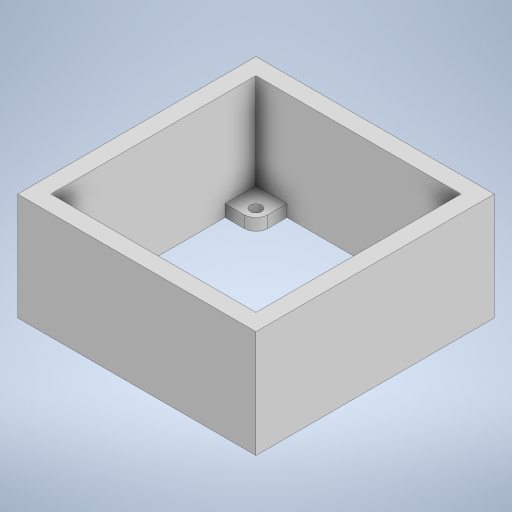
# Autodesk Inventor part: BigMotorDerzavka
Saved by Autodesk Inventor 2024 (Build 280153000, 153)
## iProperties
Created: 2023-11-07
Part Number: BigMotorDerzavka
Material: Generic
Document SubType Name: Modeling
Designer: KirikDK
Density: 1 g/cm^3
Appearance: Default
Author: KirikDK
Autodesk Inventor part; units mm, degrees
ref_plane "YZ Plane" through (0, 0, 0) normal (1, 0, 0) x (0, 1, 0)
ref_plane "XZ Plane" through (0, 0, 0) normal (0, 1, 0) x (-1, 0, 0)
ref_plane "XY Plane" through (0, 0, 0) normal (0, 0, 1) x (1, 0, 0)
sketch "Sketch1" plane through (0, 0, 0) normal (0, 1, 0) x (-1, 0, 0)
  line L0 (49.1429, 49.1429) -> (-36.8571, 49.1429)
  line L1 (-36.8571, 49.1429) -> (-36.8571, -36.8571)
  line L2 (-36.8571, -36.8571) -> (49.1429, -36.8571)
  line L3 (49.1429, -36.8571) -> (49.1429, 49.1429)
  line L4 (52.1429, 52.1429) -> (-39.8571, 52.1429)
  line L5 (-39.8571, 52.1429) -> (-39.8571, -39.8571)
  line L6 (-39.8571, -39.8571) -> (52.1429, -39.8571)
  line L7 (52.1429, -39.8571) -> (52.1429, 52.1429)
  point P0 (0, 0)
  dimension "d0" = 86
  dimension "d1" = 86
  dimension "d2" = 92
  constraints: 16 end point, 4 parallel, 2 perpendicular, 1 horizontal, 3 other
  measures "d0" distance of L0.start L0.end
  measures "d1" distance of L2.end L0.start
  measures "d2" distance of L6.end L4.start
extrude "Extrusion1" add sketch "Sketch1" along normal blind 45 contours L3 L2 L1 L0 | L7 L6 L5 L4
shell "Shell1" thickness 3 removed faces 1 at (9.1905, 45, -9.1905)
sketch "Sketch3" plane through (-49.1429, 3, -36.8571) normal (0, 1, 0) x (1, 0, 0)
  line L0 (86, -86) -> (0, -86) projected
  line L1 (86, 0) -> (0, 0) projected
  line L2 (13, -86) -> (73, -86)
  line L3 (73, -86) -> (73, 0)
  line L4 (73, 0) -> (13, 0)
  line L5 (13, 0) -> (13, -86)
  line L6 (86, 0) -> (86, -86) projected
  line L7 (86, -73) -> (0, -73)
  line L8 (0, -73) -> (0, -13)
  line L9 (0, -13) -> (86, -13)
  line L10 (86, -13) -> (86, -73)
  line L11 (0, -86) -> (0, 0) projected
  point P0 (49.1429, -36.8571)
  point P1 (73, -73)
  point P2 (73, -13)
  point P3 (13, 0)
  point P4 (13, -13)
  point P5 (13, -73)
  point P6 (73, -86)
  dimension "d6" = 13
  dimension "d7" = 13
  dimension "d8" = 13
  dimension "d9" = 13
  constraints: 16 end point, 4 parallel, 3 point on line, 2 horizontal, 2 perpendicular
  measures "d6" distance between parallel lines of L11 L5
  measures "d7" distance between parallel lines of L0 L7
  measures "d8" distance between parallel lines of L1 L9
  measures "d9" distance between parallel lines of L6 L3
extrude "Extrusion2" cut sketch "Sketch3" against normal blind 40 contours L0 L5 L7 L3 | L7 L3 L9 L6 | L7 L5 L9 L3 | L7 L8 L9 L5 | L9 L5 L1 L3
sketch "Sketch4" plane through (-49.1429, 3, 36.1429) normal (0, 1, 0) x (1, 0, 0)
  line L0 (86, -13) -> (0, -13) projected
  line L1 (0, -13) -> (0, 73) projected
  line L2 (0, 73) -> (86, 73) projected
  line L3 (86, 73) -> (86, -13) projected
  line L4 (89, -16) -> (89, 76) projected
  line L5 (89, 76) -> (-3, 76) projected
  line L6 (-3, 76) -> (-3, -16) projected
  line L7 (-3, -16) -> (89, -16) projected
  line L8 (8.2, 64.8) -> (8.2, -4.8)
  line L9 (8.2, -4.8) -> (77.8, -4.8)
  line L10 (77.8, -4.8) -> (77.8, 64.8)
  line L11 (77.8, 64.8) -> (8.2, 64.8)
  circle A0 centre (8.2, -4.8) radius 2.4
  circle A1 centre (8.2, 64.8) radius 2.4
  circle A2 centre (77.8, -4.8) radius 2.4
  circle A3 centre (77.8, 64.8) radius 2.4
  point P0 (49.1429, 36.1429)
  dimension "d12" = 69.6
  dimension "d13" = 4.8
  dimension "d14" = 4.8
  dimension "d15" = 4.8
  dimension "d16" = 4.8
  constraints: 8 end point, 4 centre point, 4 coincident, 3 other
  measures "d12" distance of L8.start L8.end
  measures "d13" diameter of A0
  measures "d14" diameter of A1
  measures "d15" diameter of A2
  measures "d16" diameter of A3
extrude "Extrusion3" cut sketch "Sketch4" against normal blind 25 contours L11 A1 L8 | L8 A1 L11 | A0 L9 L8 | L8 L9 A0 | A3 L10 L11 | L11 L10 A3 | A2 L10 L9 | L9 L10 A2
fillet "Fillet1" radius 5 4 edges at (-36.1429, 1.5, 36.1429) (-36.1429, 1.5, -23.8571) (23.8571, 1.5, 36.1429) (23.8571, 1.5, -23.8571)
sketch "Sketch5" plane through (39.8571, 0, 52.1429) normal (1, 0, 0) x (0, 0, -1)
  line L0 (0, 0) -> (92, 0) projected
  line L1 (92, 0) -> (92, 45) projected
  line L2 (0, 45) -> (92, 45) projected
  line L3 (0, 0) -> (0, 45) projected
  point P0 (52.1429, 0)
extrude "Extrusion4" add sketch "Sketch5" along normal blind 4
sketch "Sketch6" plane through (0, 45, 0) normal (0, 1, 0) x (1, 0, 0)
  line L0 (-52.1429, 39.8571) -> (-52.1429, -52.1429) projected
  line L1 (-52.1429, -52.1429) -> (43.8571, -52.1429)
  line L2 (43.8571, -52.1429) -> (43.8571, -56.1429)
  line L3 (43.8571, -56.1429) -> (-52.1429, -56.1429)
  line L4 (-52.1429, -56.1429) -> (-52.1429, -52.1429)
  line L5 (-52.1429, 39.8571) -> (43.8571, 39.8571)
  line L6 (43.8571, 39.8571) -> (43.8571, 43.8571)
  line L7 (43.8571, 43.8571) -> (-52.1429, 43.8571)
  line L8 (-52.1429, 43.8571) -> (-52.1429, 39.8571)
  line L9 (43.8571, 39.8571) -> (43.8571, -52.1429) projected
  line L10 (-52.1429, -56.1429) -> (-56.1429, -56.1429)
  line L11 (-56.1429, -56.1429) -> (-56.1429, 43.8571)
  line L12 (-56.1429, 43.8571) -> (-52.1429, 43.8571)
  line L13 (-52.1429, 43.8571) -> (-52.1429, -56.1429)
  point P0 (0, 0)
  dimension "d22" = 4
  dimension "d23" = 4
  dimension "d26" = 4
  constraints: 24 end point, 6 parallel, 3 horizontal, 3 perpendicular, 1 point on line
  measures "d22" distance of L7.end L0.start
  measures "d23" distance of L3.end L0.end
  measures "d26" distance of L3.end L10.end
extrude "Extrusion5" add sketch "Sketch6" against normal up to surface (45 mm away) contours L8 L7 L6 L5 | L0 L4 L10 L11 L12 L8 | L1 L2 L3 L4
sketch "Sketch7" plane through (-49.1429, 3, -36.8571) normal (0, 1, 0) x (1, 0, 0)
  arc A0 (8, -13) -> (13, -8) centre (8, -8) ccw projected
  line L0 (13, -8) -> (13, 0) projected
  line L1 (13, 0) -> (0, 0) projected
  line L2 (0, 0) -> (0, -13) projected
  line L3 (0, -13) -> (8, -13) projected
  circle A1 centre (8.2, -8.2) radius 2.4 projected
  arc A2 (13, -78) -> (8, -73) centre (8, -78) ccw projected
  line L4 (8, -73) -> (0, -73) projected
  line L5 (0, -73) -> (0, -86) projected
  line L6 (0, -86) -> (13, -86) projected
  line L7 (13, -86) -> (13, -78) projected
  circle A3 centre (8.2, -77.8) radius 2.4 projected
  arc A4 (78, -73) -> (73, -78) centre (78, -78) ccw projected
  line L8 (73, -78) -> (73, -86) projected
  line L9 (73, -86) -> (86, -86) projected
  line L10 (86, -86) -> (86, -73) projected
  line L11 (86, -73) -> (78, -73) projected
  circle A5 centre (77.8, -77.8) radius 2.4 projected
  arc A6 (73, -8) -> (78, -13) centre (78, -8) ccw projected
  line L12 (78, -13) -> (86, -13) projected
  line L13 (86, -13) -> (86, 0) projected
  line L14 (86, 0) -> (73, 0) projected
  line L15 (73, 0) -> (73, -8) projected
  circle A7 centre (77.8, -8.2) radius 2.4 projected
  point P0 (49.1429, -36.8571)
extrude "Extrusion6" add sketch "Sketch7" along normal blind 2
body "Solid1"
